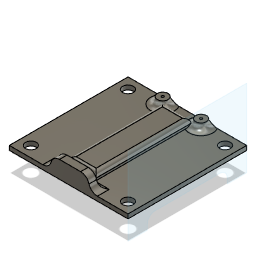
Sleep Box (Autodesk Fusion 360 design; units mm, degrees)
Autodesk Fusion 360 part; units mm, degrees
sketch "Sketch3" plane through (0, 0, 0) normal (0, 1, 0) x (1, 0, 0)
  line L0 (0, 0) -> (55, 0)
  line L1 (55, 0) -> (55, 55)
  line L2 (55, 55) -> (0, 55)
  line L3 (0, 55) -> (0, 0)
  line L4 (-1, -1) -> (56, -1)
  line L5 (56, -1) -> (56, 56)
  line L6 (56, 56) -> (-1, 56)
  line L7 (-1, 56) -> (-1, -1)
  circle A0 centre (5, 50) radius 2.5
  circle A1 centre (50, 50) radius 2.5
  circle A2 centre (5, 5) radius 2.5
  circle A3 centre (50, 5) radius 2.5
  line L8 (9, 55) -> (9, 56)
  line L9 (0, 46) -> (-1, 46)
  line L10 (46, 56) -> (46, 55)
  line L11 (56, 46) -> (55, 46)
  line L12 (0, 9) -> (-1, 9)
  line L13 (9, 0) -> (9, -1)
  line L14 (56, 9) -> (55, 9)
  line L15 (46, 0) -> (46, -1)
  dimension "d4" = 55
  dimension "d5" = 55
  dimension "d6" = 1
  dimension "d7" = 5
  dimension "d8" = 5
  dimension "d9" = 5
  dimension "d10" = 5
  dimension "d11" = 5
  dimension "d12" = 5
  dimension "d13" = 5
  dimension "d14" = 5
  dimension "d15" = 5
  dimension "d16" = 5
  dimension "d17" = 5
  dimension "d18" = 5
  dimension "d21" = 10
  dimension "d22" = 10
  dimension "d23" = 10
  dimension "d24" = 10
  dimension "d25" = 10
  dimension "d26" = 10
  dimension "d27" = 10
  dimension "d28" = 10
  constraint horizontal L0
  constraint vertical L1
  constraint horizontal L2
  constraint vertical L3
  constraint coincident L0.start L3.end
  constraint coincident L2 L8.start
  constraint coincident L6 L8.end
  constraint perpendicular L6 L8
  constraint coincident L3 L9.start
  constraint coincident L7 L9.end
  constraint perpendicular L7 L9
  constraint coincident L6 L10.start
  constraint coincident L2 L10.end
  constraint perpendicular L2 L10
  constraint coincident L5 L11.start
  constraint coincident L1 L11.end
  constraint perpendicular L1 L11
  constraint coincident L3 L12.start
  constraint coincident L7 L12.end
  constraint perpendicular L7 L12
  constraint coincident L0 L13.start
  constraint coincident L4 L13.end
  constraint perpendicular L4 L13
  constraint coincident L5 L14.start
  constraint coincident L1 L14.end
  constraint perpendicular L1 L14
  constraint coincident L0 L15.start
  constraint coincident L4 L15.end
  constraint perpendicular L4 L15
  measures "d4" distance of L0.start L0.end
  measures "d5" distance of L0.start L2.end
  measures "d7" diameter of A0
  measures "d8" distance of L2 A0.centre
  measures "d9" distance of L3 A0.centre
  measures "d10" diameter of A1
  measures "d11" distance of L2 A1.centre
  measures "d12" distance of L1 A1.centre
  measures "d13" diameter of A2
  measures "d14" distance of L3 A2.centre
  measures "d15" distance of L0 A2.centre
  measures "d16" diameter of A3
  measures "d17" distance of L1 A3.centre
  measures "d18" distance of L0 A3.centre
  measures "d21" distance of L7 L8
  measures "d22" distance of L6 L9
  measures "d23" distance of L6 L11
  measures "d24" distance of L5 L10
  measures "d25" distance of L7 L13
  measures "d26" distance of L4 L12
  measures "d27" distance of L5 L15
  measures "d28" distance of L4 L14
extrude "Extrude2" add sketch "Sketch3" along normal blind 30 contours L0 L3 L4 L7 L12 L13 | L0 L4 L13 L15 | L3 L7 L9 L12 | L0 L1 L4 L5 L14 L15 | L2 L3 L6 L7 L8 L9 | L1 L5 L11 L14 | L2 L6 L8 L10 | L1 L2 L5 L6 L10 L11 makes body 1
extrude "Extrude3" add sketch "Sketch3" against normal blind 6 contours L0 L3 L4 L7 L12 L13 | L0 L1 L4 L5 L14 L15 | L2 L3 L6 L7 L8 L9 | L1 L2 L5 L6 L10 L11 bodies 1
fillet "Fillet1" radius 3.5 8 edges at (46, 0, 0.5) (-0.5, 0, -46) (55.5, 0, -46) (46, 0, -55.5) (55.5, 0, -9) (9, 0, -55.5) (-0.5, 0, -9) (9, 0, 0.5) on bodies 1
extrude "Extrude4" add sketch "Sketch3" along normal blind 2 from surface at 3 separate body contours L0 L1 L2 L3 makes body 2
mesh "Mesh1" [no effect]
sketch "Sketch4" plane through (0, 0, -56) normal (0, 0, -1) x (-1, 0, 0)
  line L0 (-42.5, 0) -> (-12.5, 0)
  arc A0 (-9, -3.5) -> (-12.5, 0) centre (-12.5, -3.5) ccw
  line L1 (-9, -3.5) -> (-9, -6)
  line L2 (-9, -6) -> (1, -6)
  line L3 (1, -6) -> (1, 30)
  line L4 (1, 30) -> (-56, 30)
  line L5 (-56, 30) -> (-56, -6)
  line L6 (-56, -6) -> (-46, -6)
  line L7 (-46, -6) -> (-46, -3.5)
  arc A1 (-42.5, 0) -> (-46, -3.5) centre (-42.5, -3.5) ccw
  line L8 (-27.5, 0) -> (-27.5, 32) construction
  line L9 (-33, 0) -> (-33, 16)
  line L10 (-33, 16) -> (-22, 16)
  line L11 (-22, 16) -> (-22, 0)
  dimension "d37" = 16
  dimension "d38" = 11
  constraint midpoint L0 L8.start
  constraint perpendicular L0 L8
  constraint coincident L0 L9.start
  constraint perpendicular L0 L9
  constraint perpendicular L9 L10
  constraint coincident L0 L11.end
  constraint perpendicular L0 L11
  constraint midpoint L8 L10
  measures "d37" distance of L9.start L9.end
  measures "d38" distance of L9.end L10.end
extrude "Extrude5" cut sketch "Sketch4" against normal up to surface (1 mm away) contours L0 L9 L10 L11 bodies 1
fillet "Fillet2" radius 3.25 2 edges at (33, 0, -55.5) (22, 0, -55.5) on bodies 1
fillet "Fillet3" radius 1 2 edges at (22, 16, -55.5) (33, 16, -55.5) on bodies 1
sketch "Sketch5" plane through (0, 5, 0) normal (0, 1, 0) x (-1, 0, 0)
  circle A0 centre (-50, -50) radius 2.5
  circle A1 centre (-50, -5) radius 2.5
  circle A2 centre (-5, -5) radius 2.5
  circle A3 centre (-5, -50) radius 2.5
  line L0 (0, -55) -> (0, 0)
  line L1 (0, 0) -> (-55, 0)
  line L2 (-55, 0) -> (-55, -55)
  line L3 (-55, -55) -> (0, -55)
  circle A4 centre (-37.6, -6.45) radius 0.7566
  circle A5 centre (-18.2, -6.5) radius 0.9
  line L4 (-19.5, -3.5) -> (-36.7973, -3.5)
  line L5 (-36.7973, -3.5) -> (-36.7973, -0.8278)
  line L6 (-19.5, -0.8278) -> (-19.5, -3.5)
  line L7 (-19.5, 0) -> (-19.5, -0.8278)
  line L8 (-36.7973, -0.8278) -> (-36.7973, 0)
  constraint horizontal L4
  constraint vertical L5
  constraint vertical L6
  constraint coincident L1 L7.start
  constraint coincident L1 L8.end
  constraint perpendicular L1 L8
extrude "Extrude7" add sketch "Sketch5" along normal blind 6 contours L1 L4 L5 L6 L7 L8 bodies 2
fillet "Fillet5" radius 4 4 edges at (36.7973, 5, -1.75) (19.5, 5, -1.75) (19.5, 11, -1.75) (36.7973, 11, -1.75) on bodies 2
sketch "Sketch6" plane through (0, 5, 0) normal (0, 1, 0) x (-1, 0, 0)
  line L0 (-34.2333, -50) -> (-21, -50)
  line L1 (-21, -50) -> (-21, -6)
  line L2 (-21, -6) -> (-34.2333, -6)
  line L3 (-34.2333, -6) -> (-34.2333, -50)
  circle A0 centre (-18.8886, -52.1737) radius 0.55
  circle A1 centre (-18.8886, -52.1737) radius 2.5
  circle A2 centre (-36.6745, -52.1864) radius 0.55
  circle A3 centre (-36.6745, -52.1864) radius 2.5
  dimension "d66" = 1.1
  dimension "d67" = 5
  dimension "d68" = 1.1
  dimension "d69" = 5
  constraint horizontal L0
  constraint vertical L1
  constraint horizontal L2
  constraint vertical L3
  measures "d66" diameter of A0
  measures "d67" diameter of A1
  measures "d68" diameter of A2
  measures "d69" diameter of A3
extrude "Extrude9" add sketch "Sketch6" along normal blind 3 contours A0 | A1 | A2 | A3 bodies 2
extrude "Extrude8" add sketch "Sketch6" along normal blind 3 contours L0 L1 L2 L3 bodies 2
extrude "Extrude12" cut sketch "Sketch6" along normal blind 3 contours A0 bodies 2
extrude "Extrude13" cut sketch "Sketch6" along normal blind 3 contours A2 bodies 2
fillet "Fillet11" radius 3 2 edges at (21.2194, 5, -51.2696) (39.0053, 5, -51.2824) on bodies 2
sketch "Sketch7" plane through (0, 30, 0) normal (0, 1, 0) x (-1, 0, 0)
  line L0 (0, 0) -> (0, -55)
  line L1 (0, -55) -> (-55, -55)
  line L2 (-55, -55) -> (-55, 0)
  line L3 (-55, 0) -> (0, 0)
  line L4 (1, -56) -> (1, 1)
  line L5 (1, 1) -> (-56, 1)
  line L6 (-56, 1) -> (-56, -56)
  line L7 (-56, -56) -> (1, -56)
extrude "Extrude10" add sketch "Sketch7" along normal blind 1 contours L0 L1 L2 L3 | L4 L5 L6 L7 bodies 1
sketch "Sketch8" plane through (55, 0, 0) normal (-1, 0, 0) x (0, 0, 1)
  line L0 (-42.5, 0) -> (-12.5, 0)
  arc A0 (-9, -3.5) -> (-12.5, 0) centre (-12.5, -3.5) ccw
  line L1 (-9, -3.5) -> (-9, -6)
  line L2 (-9, -6) -> (0, -6)
  line L3 (0, -6) -> (0, 30)
  line L4 (0, 30) -> (-55, 30)
  line L5 (-55, 30) -> (-55, -6)
  line L6 (-55, -6) -> (-46, -6)
  line L7 (-46, -6) -> (-46, -3.5)
  arc A1 (-42.5, 0) -> (-46, -3.5) centre (-42.5, -3.5) ccw
sketch "Sketch9" plane through (55, 0, 0) normal (-1, 0, 0) x (0, 0, 1)
  line L0 (-55.617, 5.938) -> (0.383, 5.938)
  line L1 (0.383, 5.938) -> (0.383, 5.1166)
  line L2 (0.383, 5.1166) -> (-55.617, 5.1166)
  line L3 (-55.617, 5.1166) -> (-55.617, 5.938)
  dimension "d59" = 56
  constraint horizontal L0
  constraint vertical L1
  constraint horizontal L2
  constraint vertical L3
  measures "d59" distance of L0.start L0.end
extrude "Extrude11" add sketch "Sketch9" along normal blind 1 bodies 1 2
fillet "Fillet9" radius 1 1 edges at (55, 5.938, -27.5) on bodies 1
ref_plane "WorkPlane1" through (27.5, 12.5, -27.5) normal (-1, 0, 0) x (0, 0, 1)
mirror "Mirror1" about plane through (27.5, 12.5, -27.5) normal (-1, 0, 0) of "Extrude11", "Fillet9"
fillet "Fillet10" radius 2 1 edges at (28.1487, 5, -3.5) on bodies 2
fillet "Fillet12" radius 2 4 edges at (21, 8, -28) (34.2333, 8, -28) (27.6166, 8, -50) (27.6166, 8, -6) on bodies 2
hidden bodies 1
named bodies: "Housing", "Platform"
